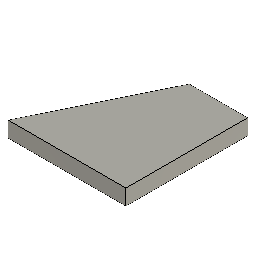
4-4 (Autodesk Fusion 360 design; units mm, degrees)
Autodesk Fusion 360 part; units mm, degrees
sketch "Sketch1" plane through (0, 0, 0) normal (0, 0, 1) x (1, 0, 0)
  line L0 (0, 0) -> (0, -600.075)
  line L1 (0, -600.075) -> (744.5375, -600.075)
  line L2 (0, 0) -> (947.7375, 0)
  line L3 (947.7375, 0) -> (744.5375, -600.075)
  line L4 (1049.3375, -600.075) -> (2105.025, -600.075)
  line L5 (1049.3375, -600.075) -> (1252.5375, 0)
  line L6 (2105.025, -600.075) -> (1698.625, 0)
  line L7 (1252.5375, 0) -> (1698.625, 0)
  line L8 (2003.425, 0) -> (3025.775, 0)
  line L9 (2409.825, -600.075) -> (3025.775, -600.075)
  line L10 (3025.775, 0) -> (3025.775, -600.075)
  line L11 (2409.825, -600.075) -> (2003.425, 0)
  line L12 (0, -904.875) -> (0, -1504.95)
  line L13 (0, -1504.95) -> (376.2375, -1504.95)
  line L14 (376.2375, -1504.95) -> (528.6375, -904.875)
  line L15 (0, -904.875) -> (528.6375, -904.875)
  line L16 (579.4375, -1504.95) -> (1636.7125, -1504.95)
  line L17 (731.8375, -904.875) -> (1420.8125, -904.875)
  line L18 (579.4375, -1504.95) -> (731.8375, -904.875)
  line L19 (1420.8125, -904.875) -> (1636.7125, -1504.95)
  line L20 (1839.9125, -1504.95) -> (2160.5875, -1504.95)
  line L21 (1624.0125, -904.875) -> (2401.8875, -904.875)
  line L22 (1624.0125, -904.875) -> (1839.9125, -1504.95)
  line L23 (2160.5875, -1504.95) -> (2401.8875, -904.875)
  line L24 (2363.7875, -1504.95) -> (3019.425, -1504.95)
  line L25 (2605.0875, -904.875) -> (3019.425, -904.875)
  line L26 (3019.425, -904.875) -> (3019.425, -1504.95)
  line L27 (2605.0875, -904.875) -> (2363.7875, -1504.95)
  line L28 (0, -1809.75) -> (0, -2409.825)
  line L29 (0, -1809.75) -> (909.6375, -1809.75)
  line L30 (0, -2409.825) -> (795.3375, -2409.825)
  line L31 (795.3375, -2409.825) -> (909.6375, -1809.75)
  line L32 (1214.4375, -1809.75) -> (2017.7125, -1809.75)
  line L33 (1100.1375, -2409.825) -> (1878.0125, -2409.825)
  line L34 (1100.1375, -2409.825) -> (1214.4375, -1809.75)
  line L35 (1878.0125, -2409.825) -> (2017.7125, -1809.75)
  line L36 (2182.8125, -2409.825) -> (3028.95, -2409.825)
  line L37 (2322.5125, -1809.75) -> (3028.95, -1809.75)
  line L38 (2322.5125, -1809.75) -> (2182.8125, -2409.825)
  line L39 (3028.95, -1809.75) -> (3028.95, -2409.825)
  line L40 (0, -2714.625) -> (0, -3314.7)
  line L41 (0, -2714.625) -> (465.1375, -2714.625)
  line L42 (465.1375, -2714.625) -> (465.1375, -3314.7)
  line L43 (465.1375, -3314.7) -> (0, -3314.7)
  line L44 (668.3375, -3314.7) -> (1268.4125, -3314.7)
  line L45 (668.3375, -3314.7) -> (668.3375, -2714.625)
  line L46 (668.3375, -2714.625) -> (1458.9125, -2714.625)
  line L47 (1458.9125, -2714.625) -> (1268.4125, -3314.7)
  line L48 (1471.6125, -3314.7) -> (2236.7875, -3314.7)
  line L49 (1662.1125, -2714.625) -> (2528.8875, -2714.625)
  line L50 (1471.6125, -3314.7) -> (1662.1125, -2714.625)
  line L51 (2528.8875, -2714.625) -> (2236.7875, -3314.7)
  line L52 (2439.9875, -3314.7) -> (3019.425, -3314.7)
  line L53 (2732.0875, -2714.625) -> (3019.425, -2714.625)
  line L54 (2439.9875, -3314.7) -> (2732.0875, -2714.625)
  line L55 (3019.425, -2714.625) -> (3019.425, -3314.7)
  dimension "d1" = 600.075
  dimension "d2" = 744.5375
  dimension "d3" = 1055.6875
  dimension "d4" = 304.8
  dimension "d5" = 1022.35
  dimension "d6" = 615.95
  dimension "d7" = 0
  dimension "d8" = 304.8
  dimension "d9" = 376.2375
  dimension "d10" = 1057.275
  dimension "d11" = 203.2
  dimension "d12" = 688.975
  dimension "d13" = 320.675
  dimension "d14" = 777.875
  dimension "d15" = 203.2
  dimension "d16" = 655.6375
  dimension "d17" = 414.3375
  dimension "d18" = 203.2
  dimension "d19" = 0
  dimension "d20" = 0
  dimension "d21" = 909.6375
  dimension "d22" = 795.3375
  dimension "d23" = 803.275
  dimension "d24" = 777.875
  dimension "d25" = 304.8
  dimension "d26" = 846.1375
  dimension "d27" = 304.8
  dimension "d28" = 706.4375
  dimension "d29" = 304.8
  dimension "d30" = 947.7375
  dimension "d31" = 446.0875
  dimension "d32" = 528.6375
  dimension "d33" = 0
  dimension "d34" = 0
  dimension "d35" = 465.1375
  dimension "d36" = 600.075
  dimension "d37" = 203.2
  dimension "d38" = 790.575
  dimension "d39" = 765.175
  dimension "d40" = 203.2
  dimension "d41" = 866.775
  dimension "d42" = 579.4375
  dimension "d43" = 287.3375
  dimension "d44" = 203.2
  constraint coincident L0.start L2.start
  constraint vertical L0
  constraint perpendicular L0 L1
  constraint perpendicular L0 L2
  constraint parallel L1 L4
  constraint parallel L3 L5
  constraint horizontal L2.end L5.end
  constraint horizontal L2.end L6.end
  constraint parallel L7 L8
  constraint collinear L7 L8
  constraint parallel L4 L9
  constraint perpendicular L9 L10
  constraint coincident L9.end L10.end
  constraint collinear L4 L9
  constraint perpendicular L1 L12
  constraint collinear L0 L12
  constraint perpendicular L12 L13
  constraint horizontal L15
  constraint parallel L13 L16
  constraint collinear L13 L16
  constraint parallel L15 L17
  constraint collinear L15 L17
  constraint parallel L14 L18
  constraint horizontal L20
  constraint collinear L16 L20
  constraint parallel L17 L21
  constraint collinear L17 L21
  constraint parallel L19 L22
  constraint parallel L20 L24
  constraint parallel L21 L25
  constraint collinear L21 L25
  constraint collinear L20 L24
  constraint parallel L23 L27
  constraint perpendicular L13 L28
  constraint perpendicular L28 L29
  constraint perpendicular L28 L30
  constraint collinear L12 L28
  constraint parallel L29 L32
  constraint parallel L30 L33
  constraint collinear L29 L32
  constraint collinear L30 L33
  constraint parallel L31 L34
  constraint parallel L33 L36
  constraint parallel L32 L37
  constraint collinear L32 L37
  constraint collinear L33 L36
  constraint parallel L35 L38
  constraint collinear L1 L4
  constraint perpendicular L30 L40
  constraint collinear L28 L40
  constraint perpendicular L40 L41
  constraint perpendicular L41 L42
  constraint perpendicular L40 L43
  constraint perpendicular L42 L44
  constraint collinear L43 L44
  constraint perpendicular L41 L45
  constraint perpendicular L42 L46
  constraint collinear L41 L46
  constraint parallel L44 L48
  constraint collinear L44 L48
  constraint parallel L46 L49
  constraint collinear L46 L49
  constraint parallel L47 L50
  constraint parallel L48 L52
  constraint collinear L48 L52
  constraint horizontal L53
  constraint collinear L49 L53
  constraint parallel L51 L54
  measures "d1" distance of L0.start L0.end
  measures "d2" distance of L0.end L1.end
  measures "d3" distance of L4.start L4.end
  measures "d4" distance of L1.end L4.start
  measures "d5" distance of L8.start L8.end
  measures "d6" distance of L9.start L9.end
  measures "d7" distance of L12.start L12.end
  measures "d8" distance of L0.end L12.start
  measures "d9" distance of L12.end L13.end
  measures "d10" distance of L16.start L16.end
  measures "d11" distance of L13.end L16.start
  measures "d12" distance of L17.start L17.end
  measures "d13" distance of L20.start L20.end
  measures "d14" distance of L21.start L21.end
  measures "d15" distance of L16.end L20.start
  measures "d16" distance of L24.start L24.end
  measures "d17" distance of L25.start L25.end
  measures "d18" distance of L20.end L24.start
  measures "d19" distance of L28.start L28.end
  measures "d20" distance of L12.end L28.start
  measures "d21" distance of L28.start L29.end
  measures "d22" distance of L28.end L30.end
  measures "d23" distance of L32.start L32.end
  measures "d24" distance of L33.start L33.end
  measures "d25" distance of L30.end L33.start
  measures "d26" distance of L36.start L36.end
  measures "d27" distance of L33.end L36.start
  measures "d28" distance of L37.start L37.end
  measures "d29" distance of L4.end L9.start
  measures "d30" distance of L0.start L2.end
  measures "d31" distance of L5.end L6.end
  measures "d32" distance of L12.start L14.end
  measures "d33" distance of L28.end L40.start
  measures "d34" distance of L40.start L40.end
  measures "d35" distance of L40.end L42.end
  measures "d36" distance of L44.start L44.end
  measures "d37" distance of L42.end L44.start
  measures "d38" distance of L45.end L46.end
  measures "d39" distance of L48.start L48.end
  measures "d40" distance of L44.end L48.start
  measures "d41" distance of L49.start L49.end
  measures "d42" distance of L52.start L52.end
  measures "d43" distance of L53.start L53.end
  measures "d44" distance of L48.end L52.start
extrude "Extrude1" add sketch "Sketch1" along normal blind 76.2 contours L52 L53 L54 L55
equation "d1 = 23 5/8\""
equation "d2 = 29 5/16\""
equation "d3 = 41 9/16\""
equation "d5 = 40 1/4\""
equation "d6 = 24 1/4\""
equation "d7 = d20"
equation "d9 = 14 13/16\""
equation "d12 = 27 1/8\""
equation "d13 = 12 5/8\""
equation "d14 = 30 5/8\""
equation "d16 = 25 13/16\""
equation "d17 = 16 5/16\""
equation "d19 = d20"
equation "d20 = d33"
equation "d21 = 35 13/16\""
equation "d22 = 31 5/16\""
equation "d23 = 31 5/8\""
equation "d24 = 30 5/8\""
equation "d26 = 33 5/16\""
equation "d28 = 27 13/16\""
equation "d30 = 37 5/16\""
equation "d31 = 17 9/16\""
equation "d32 = 20 13/16\""
equation "d33 = d33"
equation "d34 = d20"
equation "d35 = 18 5/16\""
equation "d36 = 23 5/8\""
equation "d38 = 31 1/8\""
equation "d41 = 34 1/8\""
